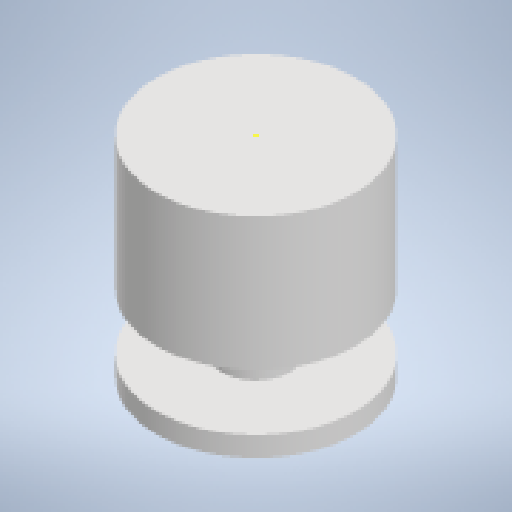
# Autodesk Inventor part: pallet
Saved by Autodesk Inventor 2023.1 (Build 271208000, 208)
## iProperties
Created: 2022-11-17
Part Number: pallet
Material: Generic
Document SubType Name: Modeling
Designer: techv
Density: 1 g/cm^3
Appearance: Default
Author: techv
Autodesk Inventor part; units mm, degrees
ref_plane "YZ Plane" through (0, 0, 0) normal (1, 0, 0) x (0, 1, 0)
ref_plane "XZ Plane" through (0, 0, 0) normal (0, 1, 0) x (-1, 0, 0)
ref_plane "XY Plane" through (0, 0, 0) normal (0, 0, 1) x (1, 0, 0)
sketch "Sketch1" plane through (0, 0, 0) normal (1, 0, 0) x (0, 1, 0)
  line L0 (-12.7, 6.35) -> (12.7, 6.35)
  line L1 (12.7, 6.35) -> (12.7, -6.35)
  line L2 (12.7, -6.35) -> (-12.7, -6.35)
  line L3 (-12.7, -6.35) -> (-12.7, 6.35)
  line L4 (-12.7, 6.35) -> (12.7, -6.35) construction
  line L5 (12.7, 6.35) -> (-12.7, -6.35) construction
  line L6 (-14.605, 19.05) -> (-10.795, 19.05)
  line L7 (-10.795, 19.05) -> (-10.795, -19.05)
  line L8 (-10.795, -19.05) -> (-14.605, -19.05)
  line L9 (-14.605, -19.05) -> (-14.605, 19.05)
  line L10 (-14.605, 19.05) -> (-10.795, -19.05) construction
  line L11 (-10.795, 19.05) -> (-14.605, -19.05) construction
  line L12 (0, 19.05) -> (25.4, 19.05)
  line L13 (25.4, 19.05) -> (25.4, -19.05)
  line L14 (25.4, -19.05) -> (0, -19.05)
  line L15 (0, -19.05) -> (0, 19.05)
  line L16 (0, 19.05) -> (25.4, -19.05) construction
  line L17 (25.4, 19.05) -> (0, -19.05) construction
  line L18 (-14.605, 0) -> (25.4, 0)
  point P0 (0, 0)
  point P1 (-12.7, 0)
  point P2 (12.7, 0)
  point P3 (-10.795, -6.35)
  point P4 (0, -6.35)
  dimension "d0" = 25.4
  dimension "d1" = 38.1
  dimension "d2" = 3.81
  dimension "d3" = 38.1
  dimension "d5" = 25.4
  dimension "d6" = 12.7
  constraints: 38 end point, 10 midpoint, 6 parallel, 3 horizontal, 3 perpendicular
  measures "d0" distance of L13.end L14.end
  measures "d1" distance of L14.end L12.start
  measures "d2" distance of L7.end L8.end
  measures "d3" distance of L8.end L6.start
  measures "d5" distance of L1.end L2.end
  measures "d6" distance of L2.end L0.start
revolve "Revolution1" add sketch "Sketch1" angle 360 about axis through (0, -14.605, 0) along (0, 1, 0) contours L18 L7 L2 L3 | L3 L2 L7 L8 L9 L18 | L18 L15 L2 L7 | L18 L1 L2 L15 | L18 L13 L14 L15 L2 L1
sketch "Sketch2" plane through (0, 25.4, 0) normal (0, 1, 0) x (1, 0, 0)
  point P0 (0, 0)
body "Solid1"
